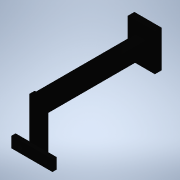
# Autodesk Inventor part: LickModuleMount_Training
Saved by Autodesk Inventor 2020 (Build 240168000, 168)
## iProperties
Created: 2019-08-06
Part Number: LickModuleMount_Training
Material: 일반
Document SubType Name: Modeling
Designer: Jeong Ji Hoon
Density: 1 g/cm^3
Appearance: 기본값
Author: Jeong Ji Hoon
## iProperties of the stored document _3D 인쇄.ipt
Created: 2019-08-06
Part Number: _3D 인쇄
Material: 일반
Document SubType Name: Modeling
Designer: Jeong Ji Hoon
Density: 1 g/cm^3
Appearance: 기본값
Author: Jeong Ji Hoon
Autodesk Inventor part; units mm, degrees
ref_plane "YZ Plane" through (0, 0, 0) normal (1, 0, 0) x (0, 1, 0)
ref_plane "XZ Plane" through (0, 0, 0) normal (0, 1, 0) x (-1, 0, 0)
ref_plane "XY Plane" through (0, 0, 0) normal (0, 0, 1) x (1, 0, 0)
sketch "스케치1" plane through (0, 0, 0) normal (0, 0, 1) x (1, 0, 0)
  line L0 (0, 0) -> (20, 0)
  line L1 (20, 0) -> (20, 27)
  line L2 (20, 27) -> (0, 27)
  line L3 (0, 27) -> (0, 0)
  dimension "d0" = 20
  dimension "d1" = 27
  constraints: 8 end point, 2 parallel, 1 horizontal, 1 perpendicular
  measures "d0" distance of L2.end L1.end
  measures "d1" distance of L1.end L0.end
extrude "돌출1" add sketch "스케치1" along normal blind 5
sketch "스케치2" plane through (0, 0, 5) normal (0, 0, 1) x (1, 0, 0)
  line L0 (0, 27) -> (0, 0) projected
  line L1 (20, 27) -> (0, 27) projected
  line L2 (6, 18.5) -> (14, 18.5)
  line L3 (14, 18.5) -> (14, 8.5)
  line L4 (14, 8.5) -> (6, 8.5)
  line L5 (6, 8.5) -> (6, 18.5)
  point P0 (6, 13.5)
  point P1 (0, 13.5)
  point P2 (10, 18.5)
  point P3 (10, 27)
  dimension "d4" = 8
  dimension "d5" = 10
  constraints: 8 end point, 4 midpoint, 2 parallel, 1 horizontal, 1 horizontal alignment, 1 perpendicular, 1 vertical alignment
  measures "d4" distance of L3.end L4.end
  measures "d5" distance of L2.end L3.end
extrude "돌출2" add sketch "스케치2" along normal blind 73
sketch "스케치3" plane through (0, 0, 78) normal (0, 0, 1) x (1, 0, 0)
  line L0 (14, 18.5) -> (6, 18.5) projected
  line L1 (5, 18.5) -> (15, 18.5)
  line L2 (15, 18.5) -> (15, -21.5)
  line L3 (15, -21.5) -> (5, -21.5)
  line L4 (5, -21.5) -> (5, 18.5)
  point P0 (0, 0)
  point P1 (10, 18.5)
  dimension "d8" = 10
  dimension "d9" = 40
  constraints: 8 end point, 2 midpoint, 2 parallel, 1 horizontal, 1 perpendicular
  measures "d8" distance of L1.start L1.end
  measures "d9" distance of L1.end L2.end
extrude "돌출3" add sketch "스케치3" along normal blind 4
sketch "스케치4" plane through (0, 0, 82) normal (0, 0, 1) x (1, 0, 0)
  line L0 (5, 18.5) -> (5, -21.5) projected
  line L1 (5, -21.5) -> (15, -21.5) projected
  line L2 (15, -21.5) -> (15, 18.5) projected
  line L3 (5, -21.5) -> (15, -21.5)
  line L4 (15, -21.5) -> (15, -11.5)
  line L5 (15, -11.5) -> (5, -11.5)
  line L6 (5, -11.5) -> (5, -21.5)
  point P0 (0, 0)
  dimension "d14" = 10
  constraints: 8 end point, 2 parallel, 1 horizontal, 1 perpendicular, 1 point on line
  measures "d14" distance between parallel lines of L1 L5
extrude "돌출4" add sketch "스케치4" along normal blind 3
sketch "스케치6" plane through (0, 0, 85) normal (0, 0, 1) x (1, 0, 0)
  line L0 (15, -21.5) -> (15, -11.5) projected
  line L1 (15, -11.5) -> (5, -11.5) projected
  line L2 (5, -11.5) -> (5, -21.5) projected
  line L3 (5, -21.5) -> (15, -21.5) projected
  line L4 (-5, -21.5) -> (25, -21.5)
  line L5 (25, -21.5) -> (25, -11.5)
  line L6 (25, -11.5) -> (-5, -11.5)
  line L7 (-5, -11.5) -> (-5, -21.5)
  point P0 (0, 0)
  point P1 (10, -11.5)
  point P2 (10, -21.5)
  point P3 (15, -21.5)
  point P4 (5, -21.5)
  point P5 (5, -11.5)
  dimension "d20" = 30
  constraints: 8 end point, 4 midpoint, 2 parallel, 1 horizontal, 1 perpendicular
  measures "d20" distance between parallel lines of L5 L7
extrude "돌출6" add sketch "스케치6" against normal blind 3 contours L0 L6 L5 L4 | L4 L7 L6 L2
sketch "스케치7" plane through (0, 0, 85) normal (0, 0, 1) x (1, 0, 0)
  line L0 (25, -11.5) -> (-5, -11.5) projected
  line L1 (-5, -11.5) -> (-5, -21.5) projected
  line L2 (25, -21.5) -> (25, -11.5) projected
  point P0 (0.75, -15.5)
  point P1 (19.25, -15.5)
  dimension "d23" = 5.75
  dimension "d24" = 4
  dimension "d25" = 5.75
  constraints: 1 horizontal alignment
  measures "d23" distance from line of L1 point (0.75, -15.5)
  measures "d24" distance from line of point (0.75, -15.5) L0
  measures "d25" distance from line of L2 point (19.25, -15.5)
hole "구멍1" at (0.75, -15.5, 85) at (19.25, -15.5, 85) direction (0, 0, -1) diameter 4 depth 4 tip angle 118
sketch "스케치8" plane through (5, -21.5, 78) normal (0, -1, 0) x (1, 0, 0)
  line L0 (0, 0) -> (10, 0) projected
  line L1 (10, 0) -> (10, 4) projected
  line L2 (20, 4) -> (10, 4) projected
  line L3 (20, 7) -> (20, 4) projected
  line L4 (-10, 7) -> (20, 7) projected
  line L5 (-10, 7) -> (-10, 4) projected
  line L6 (0, 4) -> (-10, 4) projected
  line L7 (0, 0) -> (0, 4) projected
  point P0 (-5, -78)
extrude "돌출7" cut sketch "스케치8" against normal blind 2
